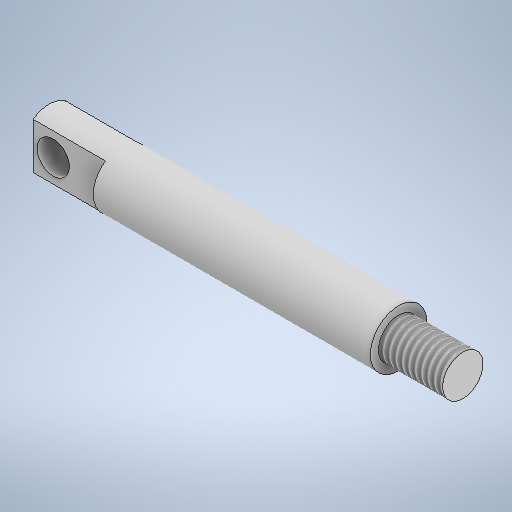
# Autodesk Inventor part: 11 fitting
Saved by Autodesk Inventor 2025.1 (Build 291241000, 241)
## iProperties
Created: 2024-09-12
Part Number: 11 fitting
Material: Generisch
Document SubType Name: Modeling
Designer: ffogue
Density: 1 g/cm^3
Appearance: Vorgabe
Author: ffogue
Autodesk Inventor part; units mm, degrees
ref_plane "YZ Plane" through (0, 0, 0) normal (1, 0, 0) x (0, 1, 0)
ref_plane "XZ Plane" through (0, 0, 0) normal (0, 1, 0) x (-1, 0, 0)
ref_plane "XY Plane" through (0, 0, 0) normal (0, 0, 1) x (1, 0, 0)
sketch "Sketch1" plane through (0, 0, 0) normal (0, 0, 1) x (1, 0, 0)
  line L0 (0, 0) -> (0, 2.5)
  line L1 (0, 2.5) -> (-8, 2.5)
  line L2 (-8, 2.5) -> (-8, 3.5)
  line L3 (-8, 3.5) -> (-51.5, 3.5)
  line L4 (-51.5, 3.5) -> (-51.5, 0)
  line L5 (-51.5, 0) -> (0, 0)
  point P0 (-4, 2.5)
  dimension "d0" = 5
  dimension "d1" = 7
  dimension "d2" = 8
  dimension "d19" = 43.5
  constraints: 12 end point, 3 perpendicular, 2 parallel, 1 midpoint, 1 vertical
  measures "d0" diameter of point (-4, 2.5) L5
  measures "d1" diameter of L3 L5
  measures "d2" distance of L0.end L1.end
  measures "d19" distance of L2.end L3.end
revolve "Revolution1" add sketch "Sketch1" angle 360 about axis through (-51.5, 0, 0) along (1, 0, 0)
thread "Thread1" size "M5x0.8" class "6g" standard "ISO Metric profile" full length
sketch "Sketch3" plane through (-51.5, 0, 0) normal (-1, 0, 0) x (0, 0, 1)
  circle A0 centre (0, 0) radius 3.5 projected
  line L0 (-2.8723, 2) -> (2.8723, 2)
  circle A1 centre (0, 0) radius 3.5 projected
  line L1 (-2.8723, -2) -> (2.8723, -2)
  arc A2 (-2.8723, 2) -> (-2.8723, -2) centre (0, 0) ccw
  arc A3 (2.8723, -2) -> (2.8723, 2) centre (0, 0) ccw
  point P0 (0, 0)
  dimension "d7" = 2
  dimension "d8" = 2
  constraints: 8 point on circle, 4 end point, 3 concentric, 2 centre point, 1 horizontal, 1 parallel, 2 other
  measures "d7" distance from line of point (0, 0) L0
  measures "d8" distance from line of L1 point (0, 0)
extrude "Extrusion1" cut sketch "Sketch3" against normal blind 9 contours L0 A0 | A0 L1
sketch "Sketch4" plane through (-51.5, -2, -2.8723) normal (0, -1, 0) x (1, 0, 0)
  line L0 (0, 0) -> (0, 5.7446) projected
  point P0 (51.5, 2.8723)
  point P1 (2.5, 2.8723)
  point P2 (0, 2.8723)
  dimension "d11" = 2.5
  constraints: 1 horizontal alignment, 1 midpoint
  measures "d11" distance from line of L0 point (2.5, 2.872)
hole "Hole1" at (-49, -2, 0) direction (0, 1, 0) diameter 4 depth 4
equation "\"d8\" = d7"
body "Solid1"
